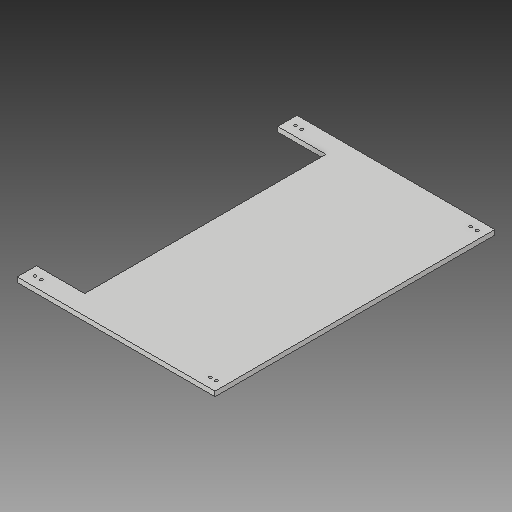
# Autodesk Inventor part: étage
Saved by Autodesk Inventor 2019 (Build 230136000, 136)
## iProperties
Created: 2019-03-31
Part Number: étage
Material: Generic
Document SubType Name: Modeling
Designer: franc
Density: 1 g/cm^3
Appearance: Default
Author: franc
Autodesk Inventor part; units mm, degrees
ref_plane "YZ Plane" through (0, 0, 0) normal (1, 0, 0) x (0, 1, 0)
ref_plane "XZ Plane" through (0, 0, 0) normal (0, 1, 0) x (-1, 0, 0)
ref_plane "XY Plane" through (0, 0, 0) normal (0, 0, 1) x (1, 0, 0)
sketch "Esquisse1" plane through (0, 0, 0) normal (0, 1, 0) x (-1, 0, 0)
  line L0 (138.2405, 132.2434) -> (-66.7595, 132.2434)
  line L1 (-66.7595, 132.2434) -> (-66.7595, -157.7566)
  line L2 (-66.7595, -157.7566) -> (138.2405, -157.7566)
  line L3 (138.2405, -157.7566) -> (138.2405, 132.2434)
  point P0 (0, 0)
  dimension "d0" = 290
  dimension "d1" = 205
  constraints: 8 end point, 2 parallel, 1 horizontal, 1 perpendicular
  measures "d0" distance of L0.end L1.end
  measures "d1" distance of L1.end L2.end
extrude "Extrusion1" add sketch "Esquisse1" along normal blind 5
sketch "Esquisse2" plane through (0, 5, 0) normal (0, 1, 0) x (1, 0, 0)
  line L0 (-138.2405, 157.7566) -> (-138.2405, -132.2434) projected
  line L1 (-138.2405, -112.2434) -> (-88.2405, -112.2434)
  line L2 (-88.2405, -112.2434) -> (-88.2405, 137.7566)
  line L3 (-88.2405, 137.7566) -> (-138.2405, 137.7566)
  line L4 (-138.2405, 137.7566) -> (-138.2405, -112.2434)
  line L5 (-138.2405, -132.2434) -> (66.7595, -132.2434) projected
  line L6 (66.7595, 157.7566) -> (-138.2405, 157.7566) projected
  point P0 (0, 0)
  dimension "d4" = 20
  dimension "d5" = 20
  dimension "d6" = 50
  constraints: 8 end point, 2 parallel, 1 horizontal, 1 perpendicular, 1 point on line
  measures "d4" distance between parallel lines of L5 L1
  measures "d5" distance between parallel lines of L6 L3
  measures "d6" distance between parallel lines of L0 L2
extrude "Extrusion2" cut sketch "Esquisse2" against normal up to next
sketch "Esquisse3" plane through (0, 5, 0) normal (0, 1, 0) x (1, 0, 0)
  circle A0 centre (58.2595, 147.7566) radius 1.5 projected
  circle A1 centre (51.7595, 147.7566) radius 1.5 projected
  circle A2 centre (58.2595, -122.2434) radius 1.5 projected
  circle A3 centre (51.7595, -122.2434) radius 1.5 projected
  circle A4 centre (-123.2405, -122.2434) radius 1.5 projected
  circle A5 centre (-129.7405, -122.2434) radius 1.5 projected
  circle A6 centre (-123.2405, 147.7566) radius 1.5 projected
  circle A7 centre (-129.7405, 147.7566) radius 1.5 projected
  point P0 (0, 0)
extrude "Extrusion3" cut sketch "Esquisse3" against normal up to next
